Autodesk Fusion 360 part; units mm, degrees
(part 2 of 2)
  spline S17 degree 5 poles (-26.3381, 19.8822) (-26.332, 19.856) (-26.3196, 19.8035) (-26.3007, 19.725) (-26.2752, 19.6205) (-26.2424, 19.4904) (-26.2089, 19.3607) (-26.1746, 19.2316) (-26.1395, 19.1029) (-26.1037, 18.9746) (-26.067, 18.8469) (-26.0296, 18.7196) (-25.9913, 18.5928) (-25.9523, 18.4666) (-25.9125, 18.3409) (-25.8719, 18.2157) (-25.8306, 18.091) (-25.7884, 17.9669) (-25.7455, 17.8433) (-25.7017, 17.7203) (-25.6572, 17.5978) (-25.6119, 17.4759) (-25.5658, 17.3546) (-25.5188, 17.2339) (-25.4711, 17.1138) (-25.4226, 16.9942) (-25.3733, 16.8754) (-25.3232, 16.7571) (-25.2723, 16.6395) (-25.2206, 16.5225) (-25.1681, 16.4061) (-25.1148, 16.2905) (-25.0607, 16.1755) (-25.0058, 16.0612) (-24.95, 15.9476) (-24.8935, 15.8348) (-24.8361, 15.7226) (-24.7779, 15.6112) (-24.7189, 15.5005) (-24.6591, 15.3906) (-24.5984, 15.2815) (-24.5369, 15.1732) (-24.4746, 15.0656) (-24.4114, 14.959) (-24.3473, 14.8531) (-24.2824, 14.7482) (-24.2167, 14.644) (-24.1501, 14.5408) (-24.0827, 14.4384) (-24.0144, 14.3369) (-23.9452, 14.2364) (-23.8751, 14.1369) (-23.8041, 14.0385) (-23.7321, 13.9412) (-23.6591, 13.845) (-23.5852, 13.7499) (-23.5105, 13.6558) (-23.4349, 13.5626) (-23.3585, 13.4705) (-23.2811, 13.3795) (-23.2027, 13.2899) (-23.1229, 13.2019) (-23.0418, 13.1158) (-22.9593, 13.0316) (-22.8756, 12.949) (-22.7909, 12.8677) (-22.7055, 12.7874) (-22.6196, 12.708) (-22.5328, 12.6298) (-22.4445, 12.554) (-22.3536, 12.4819) (-22.2781, 12.4286) (-22.2194, 12.3916) (-22.1794, 12.3683) (-22.1592, 12.357) knots -1 -1 -1 -1 -1 -1 -0.98571429 -0.97142857 -0.95714286 -0.94285714 -0.92857143 -0.91428571 -0.9 -0.88571429 -0.87142857 -0.85714286 -0.84285714 -0.82857143 -0.81428571 -0.8 -0.78571429 -0.77142857 -0.75714286 -0.74285714 -0.72857143 -0.71428571 -0.7 -0.68571429 -0.67142857 -0.65714286 -0.64285714 -0.62857143 -0.61428571 -0.6 -0.58571429 -0.57142857 -0.55714286 -0.54285714 -0.52857143 -0.51428571 -0.5 -0.48571429 -0.47142857 -0.45714286 -0.44285714 -0.42857143 -0.41428571 -0.4 -0.38571429 -0.37142857 -0.35714286 -0.34285714 -0.32857143 -0.31428571 -0.3 -0.28571429 -0.27142857 -0.25714286 -0.24285714 -0.22857143 -0.21428571 -0.2 -0.18571429 -0.17142857 -0.15714286 -0.14285714 -0.12857143 -0.11428571 -0.1 -0.08571429 -0.07142857 -0.05714286 -0.04285714 -0.02857143 -0.01428571 0 0 0 0 0 0
  line L17 (-22.1592, 12.357) -> (-18.5835, 10.3615)
  arc A35 (-17.9169, 8.3075) -> (-18.5835, 10.3615) centre (-19.3572, 8.9753) ccw
  circle A36 centre (0, 0) radius 3.5
  circle A37 centre (0, 0) radius 2.85
  line L18 (0, 0) -> (0, 1.953) construction
  line L19 (0, 0) -> (0, -1.953) construction
  line L20 (0, -1.953) -> (-2.0756, -1.953)
  line L21 (0, -1.953) -> (2.0756, -1.953)
  line L22 (0, 1.953) -> (-2.0756, 1.953)
  line L23 (0, 1.953) -> (2.0756, 1.953)
  dimension "d9" = 7
  dimension "d10" = 5.7
  dimension "d11" = 1.953
  dimension "d12" = 1.953
  constraint concentric A0 A36
  constraint concentric A0 A37
  constraint coincident A0.centre A2.centre
  constraint vertical L18
  constraint parallel L18 L19
  constraint coincident A37 L20.end
  constraint perpendicular L19 L20
  constraint coincident A37 L21.end
  constraint perpendicular L19 L21
  constraint coincident A37 L22.end
  constraint perpendicular L18 L22
  constraint coincident A37 L23.end
  constraint perpendicular L18 L23
  measures "d9" diameter of A36
  measures "d10" diameter of A37
  measures "d11" distance of A0.centre L18.end
  measures "d12" distance of A0.centre L19.end
extrude "Extrude3" add sketch "Sketch1 (2)" along normal blind 10 contours A36 | A37 L22 L23 | A37 L20 L21 in component "Spur Gear (9 teeth)"
extrude "Extrude4" add 1 faces at (4.5627, -0.2983, 0) along direction (0, 0, -1) blind 5 in component "Spur Gear (9 teeth)"
extrude "Extrude5" cut 1 faces at (4.5627, -0.2983, -5) along direction (0, 0, 1) blind 5 in component "Spur Gear (9 teeth)"
component "Spur Gear (9 teeth)" placed x (1, 0, 0) y (0, 1, 0) z (0, 0, 1) at (0, 0, 0)
